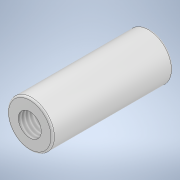
# Autodesk Inventor part: スペーサーM4L21アルミ
Saved by Autodesk Inventor 2020.2 (Build 242310000, 310)
## iProperties
Created: 2020-02-24
Part Number: スペーサーM4L21アルミ
Material: アルミニウム 2014-T4
Document SubType Name: Modeling
Designer: aoyam
Density: 2.8 g/cm^3
Appearance: サテン
Mass: 1.36366 g
Surface Area: 5.32278 cm^2
Volume: 0.48702 cm^3
Author: aoyam
Autodesk Inventor part; units mm, degrees
ref_plane "YZ Plane" through (0, 0, 0) normal (1, 0, 0) x (0, 1, 0)
ref_plane "XZ Plane" through (0, 0, 0) normal (0, 1, 0) x (-1, 0, 0)
ref_plane "XY Plane" through (0, 0, 0) normal (0, 0, 1) x (1, 0, 0)
sketch "スケッチ1" plane through (0, 0, 0) normal (0, 0, 1) x (1, 0, 0)
  circle A0 centre (0, 0) radius 4
  circle A1 centre (0, 0) radius 2
  dimension "d0" = 8
  dimension "d1" = 4
  constraints: 2 centre point, 2 coincident
  measures "d0" diameter of A0
  measures "d1" diameter of A1
extrude "押し出し1" add sketch "スケッチ1" along normal blind 21
fillet "フィレット1" radius 0.3 2 edges at (-4, 0, 21) (-4, 0, 0)
thread "ねじ1" size "M4x0.7" class "6H" standard "ANSI Metric M Profile" length 100
extrude "押し出し2" add sketch "スケッチ1" along normal blind 15 contours A1
extrude "押し出し3" cut sketch "スケッチ1" along normal blind 6 contours A1
thread "ねじ2" size "M4x0.7" class "6H" standard "ANSI Metric M Profile" full length
